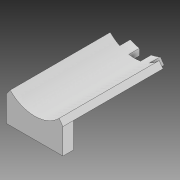
# Autodesk Inventor part: 2103_Tx_CoilFin_Spacer_V1
Saved by Autodesk Inventor 2021 (Build 250183000, 183)
## iProperties
Created: 2022-08-11
Part Number: 2103_Tx_CoilFin_Spacer_V1
Material: Generic
Document SubType Name: Modeling
Designer: Eli
Density: 1 g/cm^3
Appearance: Default
Author: Eli
Autodesk Inventor part; units mm, degrees
ref_plane "YZ Plane" through (0, 0, 0) normal (1, 0, 0) x (0, 1, 0)
ref_plane "XZ Plane" through (0, 0, 0) normal (0, 1, 0) x (-1, 0, 0)
ref_plane "XY Plane" through (0, 0, 0) normal (0, 0, 1) x (1, 0, 0)
sketch "Sketch1" plane through (0, 0, 0) normal (0, 0, 1) x (1, 0, 0)
  circle A0 centre (0, 0) radius 19
  circle A1 centre (0, 0) radius 16
  line L0 (0, 0) -> (0, -16) construction
  line L1 (-2.75, 14) -> (2.75, 14)
  line L2 (2.75, 14) -> (2.75, 19)
  line L3 (2.75, 19) -> (-2.75, 19)
  line L4 (-2.75, 19) -> (-2.75, 14)
  line L5 (-10.4538, 9.7098) -> (-6.0042, 12.9426)
  line L6 (-6.0042, 12.9426) -> (-8.9431, 16.9877)
  line L7 (-13.3927, 13.7549) -> (-10.4538, 9.7098)
  line L8 (-8.9431, 16.9877) -> (-13.3927, 13.7549)
  line L9 (-14.1646, 1.7108) -> (-12.465, 6.9416)
  line L10 (-12.465, 6.9416) -> (-17.2203, 8.4867)
  line L11 (-18.9199, 3.2559) -> (-14.1646, 1.7108)
  line L12 (-17.2203, 8.4867) -> (-18.9199, 3.2559)
  line L13 (-12.465, -6.9416) -> (-14.1646, -1.7108)
  line L14 (-14.1646, -1.7108) -> (-18.9199, -3.2559)
  line L15 (-17.2203, -8.4867) -> (-12.465, -6.9416)
  line L16 (-18.9199, -3.2559) -> (-17.2203, -8.4867)
  line L17 (-6.0042, -12.9426) -> (-10.4538, -9.7098)
  line L18 (-10.4538, -9.7098) -> (-13.3927, -13.7549)
  line L19 (-8.9431, -16.9877) -> (-6.0042, -12.9426)
  line L20 (-13.3927, -13.7549) -> (-8.9431, -16.9877)
  line L21 (2.75, -14) -> (-2.75, -14)
  line L22 (-2.75, -14) -> (-2.75, -19)
  line L23 (2.75, -19) -> (2.75, -14)
  line L24 (-2.75, -19) -> (2.75, -19)
  line L25 (10.4538, -9.7098) -> (6.0042, -12.9426)
  line L26 (6.0042, -12.9426) -> (8.9431, -16.9877)
  line L27 (13.3927, -13.7549) -> (10.4538, -9.7098)
  line L28 (8.9431, -16.9877) -> (13.3927, -13.7549)
  line L29 (14.1646, -1.7108) -> (12.465, -6.9416)
  line L30 (12.465, -6.9416) -> (17.2203, -8.4867)
  line L31 (18.9199, -3.2559) -> (14.1646, -1.7108)
  line L32 (17.2203, -8.4867) -> (18.9199, -3.2559)
  line L33 (12.465, 6.9416) -> (14.1646, 1.7108)
  line L34 (14.1646, 1.7108) -> (18.9199, 3.2559)
  line L35 (17.2203, 8.4867) -> (12.465, 6.9416)
  line L36 (18.9199, 3.2559) -> (17.2203, 8.4867)
  line L37 (6.0042, 12.9426) -> (10.4538, 9.7098)
  line L38 (10.4538, 9.7098) -> (13.3927, 13.7549)
  line L39 (8.9431, 16.9877) -> (6.0042, 12.9426)
  line L40 (13.3927, 13.7549) -> (8.9431, 16.9877)
  point P0 (-10.6247, -15.7517)
  point P1 (10.6247, -15.7517)
  point P2 (-14.3395, -12.4651)
  point P3 (14.3395, -12.4651)
  point P4 (0, 14)
  point P5 (-8.229, 11.3262)
  point P6 (-13.3148, 4.3262)
  point P7 (-13.3148, -4.3262)
  point P8 (-8.229, -11.3262)
  point P9 (0, -14)
  point P10 (8.229, -11.3262)
  point P11 (13.3148, -4.3262)
  point P12 (13.3148, 4.3262)
  point P13 (8.229, 11.3262)
  point P14 (8.8255, -16.8259)
  point P15 (7.0398, -14.3681)
  point P16 (2.75, -15.7619)
  point P17 (2.75, -18.7999)
  point P18 (-2.75, -18.7999)
  point P19 (-2.75, -15.7619)
  point P20 (-7.0398, -14.3681)
  point P21 (-8.8255, -16.8259)
  point P22 (-11.4894, -11.1352)
  point P23 (-13.2751, -13.5931)
  point P24 (13.2751, -13.5931)
  point P25 (11.4894, -11.1352)
  dimension "d0" = 38
  dimension "d1" = 3
  dimension "d13" = 5.5
  dimension "d14" = 5
  dimension "d17" = 360
  constraints: 82 end point, 4 point on circle, 2 parallel, 1 centre point, 1 coincident, 1 horizontal, 1 midpoint, 1 perpendicular, 1 tangent, 1 vertical, 1 vertical alignment, 94 other
  measures "d0" diameter of A0
  measures "d13" distance of L3.end L2.end
  measures "d14" distance of L2.end L1.end
extrude "Extrusion4" add sketch "Sketch1" along normal blind 42 contours A0 L26 A1 L27 | L26 A0 L23 A1 | L23 A0 L22 A1 | L22 A0 L19 A1 | L19 A0 L18 A1
extrude "Extrusion5" add sketch "Sketch1" against normal blind 5 contours L26 A0 L23 A1 | L22 A0 L19 A1
sketch "Sketch3" plane through (0, 0, 42) normal (0, 0, 1) x (1, 0, 0)
  arc A0 (-11.4894, -11.1352) -> (11.4894, -11.1352) centre (0, 0) ccw projected
  line L0 (-11.4894, -11.1352) -> (-13.2751, -13.5931) projected
  arc A1 (-13.2751, -13.5931) -> (13.2751, -13.5931) centre (0, 0) ccw projected
  line L1 (13.2751, -13.5931) -> (11.4894, -11.1352) projected
  line L2 (-11.4894, -11.1352) -> (-13.2751, -13.5931) projected
  line L3 (-13.2751, -13.5931) -> (13.2751, -13.5931)
  line L4 (13.2751, -13.5931) -> (13.2751, -25.5931)
  line L5 (13.2751, -25.5931) -> (-13.2751, -25.5931)
  line L6 (-13.2751, -25.5931) -> (-13.2751, -13.5931)
  dimension "d23" = 12
  constraints: 8 end point, 2 parallel, 1 horizontal, 1 perpendicular
  measures "d23" distance of L1.start L4.end
extrude "Extrusion6" add sketch "Sketch3" along normal blind 5 contours A0 L3 L0 | A0 L3 A1 | A1 L4 L5 L6 | A0 L1 L3
body "Solid2"
